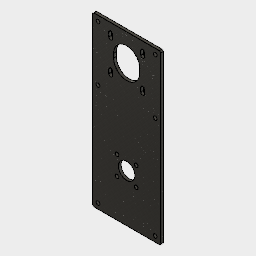
AxisTot1 (Autodesk Fusion 360 archive; units mm, degrees)
design "Axis1part2"
Autodesk Fusion 360 part; units mm, degrees
sketch "Sketch1" plane through (0, 0, 0) normal (0, 0, 1) x (1, 0, 0) in component "Axis1part2"
  line L0 (50, 123.5) -> (-50, 123.5)
  line L1 (-50, 123.5) -> (-50, -123.5)
  line L2 (-50, -123.5) -> (50, -123.5)
  line L3 (50, -123.5) -> (50, 123.5)
  line L4 (50, 123.5) -> (-50, -123.5) construction
  line L5 (-50, 123.5) -> (50, -123.5) construction
  circle A0 centre (-42, 115.5) radius 2.625
  circle A1 centre (-42, 34.5) radius 2.625
  circle A2 centre (-42, -115.5) radius 2.625
  circle A3 centre (42, -115.5) radius 2.625
  circle A4 centre (42, 34.5) radius 2.625
  circle A5 centre (42, 115.5) radius 2.625
  circle A6 centre (0, -53.5) radius 12
  circle A7 centre (14, -39.5) radius 2.625
  circle A8 centre (14, -67.5) radius 2.625
  circle A9 centre (-14, -39.5) radius 2.625
  circle A10 centre (-14, -67.5) radius 2.625
  line L6 (19.05, 80.5) -> (19.05, 86.5)
  arc A11 (19.05, 86.5) -> (-19.05, 86.5) centre (0, 86.5) ccw
  line L7 (-19.05, 86.5) -> (-19.05, 80.5)
  arc A12 (-19.05, 80.5) -> (19.05, 80.5) centre (0, 80.5) ccw
  line L8 (0, 80.5) -> (0, 86.5) construction
  line L9 (26.13, 104) -> (26.13, 110)
  arc A13 (26.13, 110) -> (20.87, 110) centre (23.5, 110) ccw
  line L10 (20.87, 110) -> (20.87, 104)
  arc A14 (20.87, 104) -> (26.13, 104) centre (23.5, 104) ccw
  line L11 (23.5, 104) -> (23.5, 110) construction
  line L12 (20.87, 63) -> (20.87, 57)
  arc A15 (20.87, 57) -> (26.13, 57) centre (23.5, 57) ccw
  line L13 (26.13, 57) -> (26.13, 63)
  arc A16 (26.13, 63) -> (20.87, 63) centre (23.5, 63) ccw
  line L14 (23.5, 63) -> (23.5, 57) construction
  line L15 (-20.87, 57) -> (-20.87, 63)
  arc A17 (-20.87, 63) -> (-26.13, 63) centre (-23.5, 63) ccw
  line L16 (-26.13, 63) -> (-26.13, 57)
  arc A18 (-26.13, 57) -> (-20.87, 57) centre (-23.5, 57) ccw
  line L17 (-23.5, 57) -> (-23.5, 63) construction
  line L18 (-26.13, 110) -> (-26.13, 104)
  arc A19 (-26.13, 104) -> (-20.87, 104) centre (-23.5, 104) ccw
  line L19 (-20.87, 104) -> (-20.87, 110)
  arc A20 (-20.87, 110) -> (-26.13, 110) centre (-23.5, 110) ccw
  line L20 (-23.5, 110) -> (-23.5, 104) construction
  line L21 (0, 123.5) -> (0, -90) construction
  line L22 (0, 83.5) -> (66.5893, 83.5) construction
  line L23 (0, -53.5) -> (63.7909, -53.5) construction
  line L24 (-42, 115.5) -> (-42, -96.5651) construction
  line L25 (42, 115.5) -> (42, -100) construction
  point P0 (0, 83.5)
  point P1 (23.5, 107)
  point P2 (23.5, 60)
  point P3 (-23.5, 60)
  point P4 (-23.5, 107)
  dimension "d1" = 100
  dimension "d2" = 247
  dimension "d5" = 19.05
  dimension "d6" = 6
  dimension "d7" = 207
  dimension "d8" = 2.63
  dimension "d9" = 23.5
  dimension "d10" = 23.5
  dimension "d11" = 5.25
  dimension "d12" = 5.25
  dimension "d13" = 24
  dimension "d14" = 70
  dimension "d15" = 28
  dimension "d16" = 28
  dimension "d17" = 8
  dimension "d18" = 8
  dimension "d19" = 8
  dimension "d20" = 158
  dimension "d21" = 8
  measures "d1" distance of L0.start L0.end
  measures "d2" distance of L0.end L1.end
  measures "d5" radius of A12
  measures "d6" distance of A12.centre A11.centre
  measures "d7" distance of L2 P0
  measures "d8" radius of A19
  measures "d9" distance of P4 L21
  measures "d10" distance of P1 L22
  measures "d11" diameter of A0
  measures "d12" diameter of A10
  measures "d13" diameter of A6
  measures "d14" distance of L2 A6.centre
  measures "d15" distance of A7.centre A9.centre
  measures "d16" distance of A7.centre A8.centre
  measures "d17" distance of L0 A0.centre
  measures "d18" distance of L1 A0.centre
  measures "d19" distance of L2 A2.centre
  measures "d20" distance of L2 A1.centre
  measures "d21" distance of L3 A5.centre
extrude "Extrude1" add sketch "Sketch1" along normal blind 4 in component "Axis1part2"
fillet "Fillet1" radius 2 4 edges at (50, 123.5, 2) (-50, 123.5, 2) (50, -123.5, 2) (-50, -123.5, 2) in component "Axis1part2"
component "Axis1part2" placed x (1, 0, 0) y (0, 1, 0) z (0, 0, 1) at (0, 0, 0)

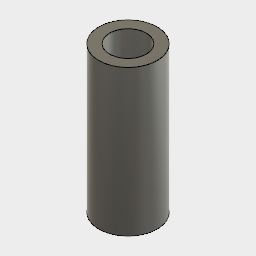
design "M5standoff"
Autodesk Fusion 360 part; units mm, degrees
sketch "Sketch1" plane through (0, 0, 0) normal (0, 1, 0) x (1, 0, 0) in component "M5standoff"
  circle A0 centre (0, 0) radius 4
  circle A1 centre (0, 0) radius 2.5
  dimension "d1" = 5
  dimension "d2" = 8
  measures "d1" diameter of A1
  measures "d2" diameter of A0
extrude "Extrude1" add sketch "Sketch1" along normal blind 20 in component "M5standoff"
component "M5standoff" placed x (1, 0, 0) y (0, 1, 0) z (0, 0, 1) at (0, 0, 0)
